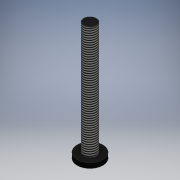
# Autodesk Inventor part: Hex Screws used in Desk
Saved by Autodesk Inventor 2016 (Build 200138000, 138)
## iProperties
Created: 2015-11-19
Part Number: Hex Screws used in Desk
Material: 常规
Document SubType Name: Modeling
Designer: Shawn Shi Feng
Density: 1 g/cm^3
Appearance: 默认
Author: Shawn Shi Feng
Autodesk Inventor part; units mm, degrees
ref_plane "YZ Plane" through (0, 0, 0) normal (1, 0, 0) x (0, 1, 0)
ref_plane "XZ Plane" through (0, 0, 0) normal (0, 1, 0) x (-1, 0, 0)
ref_plane "XY Plane" through (0, 0, 0) normal (0, 0, 1) x (1, 0, 0)
sketch "草图1" plane through (0, 0, 0) normal (0, 0, 1) x (1, 0, 0)
  circle A0 centre (0, 0) radius 2.5
  dimension "d0" = 5
  constraints: 1 centre point, 1 coincident
  measures "d0" diameter of A0
extrude "拉伸1" add sketch "草图1" along normal blind 44
sketch "草图2" plane through (0, 0, 0) normal (0, 0, -1) x (-1, 0, 0)
  circle A0 centre (0, 0) radius 5
  dimension "d3" = 10
  constraints: 1 centre point, 1 coincident
  measures "d3" diameter of A0
extrude "拉伸2" add sketch "草图2" along normal blind 2
sketch "草图3" plane through (0, 0, -2) normal (0, 0, -1) x (-1, 0, 0)
  circle A0 centre (0, 0) radius 2.5 projected
  line L0 (2.5, 0) -> (1.25, -2.1651)
  line L1 (1.25, -2.1651) -> (-1.25, -2.1651)
  line L2 (-1.25, -2.1651) -> (-2.5, 0)
  line L3 (-2.5, 0) -> (-1.25, 2.1651)
  line L4 (-1.25, 2.1651) -> (1.25, 2.1651)
  line L5 (1.25, 2.1651) -> (2.5, 0)
  dimension "d6" = 4.3301
  constraints: 12 end point, 1 coincident, 1 horizontal alignment, 14 other
  measures "d6" vertical distance of L4.end L1.end
extrude "拉伸3" cut sketch "草图3" against normal blind 2 contours L0 L1 L2 L3 L4 L5
thread "螺纹1" size "M5x0.8" class "6g" standard "ANSI Metric M Profile" full length
